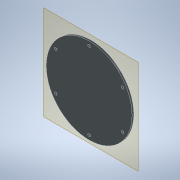
# Autodesk Inventor part: Крышка картера 4
Saved by Autodesk Inventor 2021 (Build 250183000, 183)
## iProperties
Created: 2020-12-12
Part Number: Крышка картера 4
Material: Чугун, серый
Document SubType Name: Modeling
Designer: Тимоха
Mass: 1744.09 g
Surface Area: 1022.53 cm^2
Volume: 243.929 cm^3
Density: 7.15 g/cm^3
Appearance: Чугун серый
Author: Тимоха
Autodesk Inventor part; units mm, degrees
ref_plane "YZ Plane" through (0, 0, 0) normal (1, 0, 0) x (0, 1, 0)
ref_plane "XZ Plane" through (0, 0, 0) normal (0, 1, 0) x (-1, 0, 0)
ref_plane "XY Plane" through (0, 0, 0) normal (0, 0, 1) x (1, 0, 0)
ref_plane "РабПлоскость1" through (0, 0, 0) normal (0, 0, 1) x (1, 0, 0)
sketch "Эскиз1" plane through (0, 0, 0) normal (0, 0, 1) x (1, 0, 0)
  circle A0 centre (97.4279, 56.25) radius 4 projected
  circle A1 centre (97.4279, -56.25) radius 4 projected
  circle A2 centre (0, -112.5) radius 4 projected
  circle A3 centre (-97.4279, -56.25) radius 4 projected
  circle A4 centre (-97.4279, 56.25) radius 4 projected
  circle A5 centre (0, 112.5) radius 4 projected
  circle A6 centre (0, 0) radius 125 projected
  circle A7 centre (0, 0) radius 100 projected
extrude "Выдавливание1" add sketch "Эскиз1" along normal blind 5 contours A6 | A7
